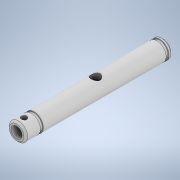
# Autodesk Inventor part: potentiometer_aksel
Saved by Autodesk Inventor 2022 (Build 260153000, 153)
## iProperties
Created: 2022-05-04
Part Number: potentiometer_aksel
Material: Generic
Document SubType Name: Modeling
Designer: Patrick
Density: 1 g/cm^3
Appearance: Default
Author: Patrick
Autodesk Inventor part; units mm, degrees
ref_plane "YZ Plane" through (0, 0, 0) normal (1, 0, 0) x (0, 1, 0)
ref_plane "XZ Plane" through (0, 0, 0) normal (0, 1, 0) x (-1, 0, 0)
sketch "Sketch1" plane through (0, 0, 0) normal (0, 1, 0) x (-1, 0, 0)
  line L0 (0, 0) -> (4.0002, 0)
  line L1 (4.0002, 0) -> (5, -0.9998)
  line L2 (5, -0.9998) -> (5, -8)
  line L3 (5, -8) -> (4.5, -8)
  line L4 (4.5, -8) -> (4.5, -9.5)
  line L5 (4.5, -9.5) -> (5, -9.5)
  line L6 (5, -9.5) -> (5, -76.5)
  line L7 (5, -76.5) -> (4.5, -76.5)
  line L8 (4.5, -76.5) -> (4.5, -78)
  line L9 (4.5, -78) -> (5, -78)
  line L10 (5, -78) -> (5, -79)
  line L11 (5, -79) -> (4, -80)
  line L12 (4, -80) -> (0, -80)
  line L13 (0, -80) -> (0, 0)
  dimension "d9" = 80
  dimension "d10" = 5
  dimension "d11" = 0.5
  dimension "d12" = 1.5
  dimension "d13" = 1.5
  dimension "d14" = 2
  dimension "d15" = 1
  dimension "d16" = 135
  dimension "d17" = 67
  dimension "d18" = 135
  dimension "d19" = 1.414
  constraints: 28 end point, 7 perpendicular, 6 point on line, 1 horizontal, 1 parallel
  measures "d9" distance of L12.end L0.start
  measures "d10" distance between parallel lines of L13 L6
  measures "d11" distance of L4.end L5.end
  measures "d12" distance of L3.end L4.end
  measures "d13" distance of L7.end L8.end
  measures "d14" distance between parallel lines of L9 L12
  measures "d15" distance of L9.end L10.end
  measures "d16" angle of L12 L11
  measures "d17" distance of L5.end L6.end
  measures "d18" angle of L1 L0
  measures "d19" distance of L0.end L1.end
revolve "Revolution1" add sketch "Sketch1" angle 360 about axis through (0, 0, -80) along (0, 0, 1)
sketch "Sketch2" plane through (0, 0, 0) normal (0, 0, 1) x (1, 0, 0)
  circle A0 centre (0, 0) radius 3
  dimension "d21" = 6
  constraints: 1 centre point, 1 coincident
  measures "d21" diameter of A0
extrude "Extrusion1" cut sketch "Sketch2" against normal blind 10
ref_plane "Work Plane1" through (0, 5, 0) normal (0, 1, 0) x (-1, 0, 0)
sketch "Sketch3" plane through (0, 5, 0) normal (0, 1, 0) x (-1, 0, 0)
  line L0 (-5, -9.5) -> (5, -9.5) projected
  line L1 (-5, -76.5) -> (5, -76.5) projected
  line L2 (-5, -9.5) -> (-5, -76.5) projected
  line L3 (5, -9.5) -> (5, -76.5) projected
  circle A0 centre (0, -43) radius 2.5
  point P0 (0, 0)
  dimension "d25" = 5
  dimension "d26" = 67
  dimension "d27" = 33.5
  constraints: 1 centre point
  measures "d25" diameter of A0
  measures "d26" distance of L2.start L2.end
  measures "d27" distance from line of A0.centre L0
extrude "Extrusion2" cut sketch "Sketch3" against normal blind 10 contours A0
sketch "Sketch4" plane through (0, 5, 0) normal (0, 1, 0) x (-1, 0, 0)
  line L0 (-5, -0.9998) -> (5, -0.9998) projected
  line L1 (-5, -8) -> (5, -8) projected
  line L2 (-5, -0.9998) -> (-5, -8) projected
  line L3 (5, -0.9998) -> (5, -8) projected
  circle A0 centre (0, -4) radius 1.5
  line L4 (-4.0002, 0) -> (4.0002, 0) projected
  point P0 (0, 0)
  dimension "d30" = 3
  dimension "d31" = 4
  constraints: 1 centre point
  measures "d30" diameter of A0
  measures "d31" distance from line of L4 A0.centre
extrude "Extrusion3" cut sketch "Sketch4" against normal up to surface contours A0
thread "Thread1" size "M3x0.5" class "6H" standard "ANSI Metric M Profile" length 10
thread "Thread2" size "M5x0.8" class "6H" standard "ANSI Metric M Profile" length 10
equation "\"d27\" = 0.5 * d26"
body "Solid1"
